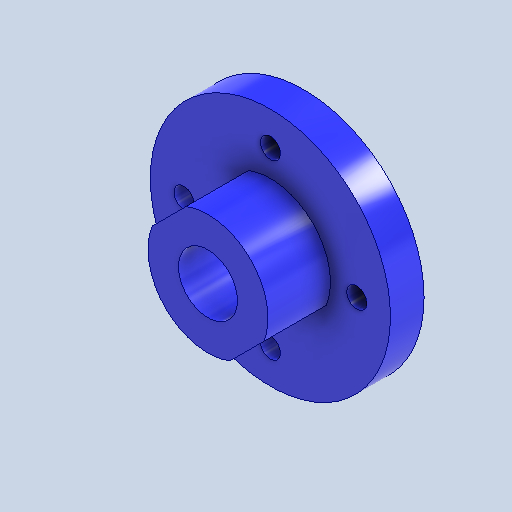
# Autodesk Inventor part: TH22_3DP_roller_fixer_sn
Saved by Autodesk Inventor 2025.1 (Build 291241000, 241)
## iProperties
Created: 2021-11-15
Part Number: TH22_3DP_roller_fixer_sn
Material: ABS プラスチック
Document SubType Name: Modeling
Designer: 中島 青蔵
Density: 1.06 g/cm^3
Appearance: 青 - 壁塗料 - 光沢
Author: 中島 青蔵
Autodesk Inventor part; units mm, degrees
ref_plane "YZ Plane" through (0, 0, 0) normal (1, 0, 0) x (0, 1, 0)
ref_plane "XZ Plane" through (0, 0, 0) normal (0, 1, 0) x (-1, 0, 0)
ref_plane "XY Plane" through (0, 0, 0) normal (0, 0, 1) x (1, 0, 0)
sketch "スケッチ1" plane through (0, 0, 0) normal (0, 0, 1) x (1, 0, 0)
  circle A0 centre (0, 0) radius 25
  circle A1 centre (0, 0) radius 6.15
  circle A2 centre (0, 0) radius 12.5
  line L0 (0, 0) -> (-8.8388, 8.8388)
  line L1 (0, 0) -> (12.5, 0) construction
  line L2 (-8.1009, 8.1009) -> (-4.5654, 11.6365)
  line L3 (-8.1009, 8.1009) -> (-11.6365, 4.5654)
  line L4 (8.1009, -8.1009) -> (4.5654, -11.6365)
  line L5 (8.1009, -8.1009) -> (11.6365, -4.5654)
  circle A3 centre (0, 18) radius 2.1
  circle A4 centre (-18, 0) radius 2.1
  circle A5 centre (0, -18) radius 2.1
  circle A6 centre (18, 0) radius 2.1
  dimension "d0" = 50
  dimension "d1" = 12.3
  dimension "d2" = 25
  dimension "d3" = 135
  dimension "d4" = 5
  dimension "d7" = 360
  dimension "d9" = 18
  dimension "d12" = 360
  dimension "d14" = 4.2
  dimension "d17" = 360
  constraints: 12 end point, 7 centre point, 4 coincident, 2 point on circle, 1 equal length, 1 horizontal, 1 perpendicular, 1 point on line, 1 symmetric about line, 25 other
  measures "d0" diameter of A0
  measures "d1" diameter of A1
  measures "d2" diameter of A2
  measures "d3" angle of L1 L0
  measures "d4" distance of L2.start L2.end
  measures "d9" distance of point (0, 0) point (0, 18)
  measures "d14" diameter of A3
extrude "押し出し1" add sketch "スケッチ1" along normal blind 7 contours A0 | L2 L0 A2 | A2 L4 L5 | L0 L3 A2
extrude "押し出し2" add sketch "スケッチ1" along normal blind 20 contours A2 L5 L4 L3 L2
sketch "スケッチ2" plane through (11.6365, -4.5654, 20) normal (0.7071068, -0.7071068, 0) x (-0.7071068, -0.7071068, 0)
  line L0 (10, 0) -> (0, 0) projected
  point P0 (5, 20)
  point P1 (5, 6.5)
  dimension "d23" = 6.5
  measures "d23" distance from line of L0 point (5, 6.5)
hole "穴1" at (8.1009, -8.1009, 13.5) direction (-0.7071068, 0.7071068, 0) diameter 4 end through all
